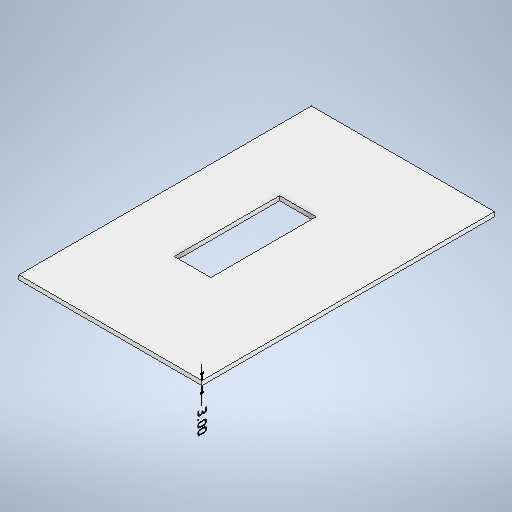
# Autodesk Inventor part: Q top 2
Saved by Autodesk Inventor 2025.3 (Build 293356000, 356)
## iProperties
Created: 2026-04-17
Part Number: Q top 2
Material: ABS Plastic
Document SubType Name: Modeling
Designer: logien
Density: 1.06 g/cm^3
Appearance: Smooth - White
Author: logien
Autodesk Inventor part; units mm, degrees
ref_plane "YZ Plane" through (0, 0, 0) normal (1, 0, 0) x (0, 1, 0)
ref_plane "XZ Plane" through (0, 0, 0) normal (0, 1, 0) x (-1, 0, 0)
ref_plane "XY Plane" through (0, 0, 0) normal (0, 0, 1) x (1, 0, 0)
sketch "Sketch1" plane through (0, 0, 0) normal (0, 1, 0) x (-1, 0, 0)
  line L0 (0, 0) -> (125.16, 0)
  line L1 (125.16, 0) -> (125.16, -200)
  line L2 (125.16, -200) -> (0, -200)
  line L3 (0, -200) -> (0, 0)
  dimension "d0" = 200
  dimension "d1" = 125.16
  constraints: 8 end point, 2 parallel, 1 horizontal, 1 perpendicular
  measures "d0" distance of L2.end L0.start
  measures "d1" distance of L0.start L0.end
extrude "Extrusion1" add sketch "Sketch1" along normal blind 3
sketch "Sketch2" plane through (0, 3, 0) normal (0, 1, 0) x (1, 0, 0)
  line L0 (-82.935, 64) -> (-57.935, 64)
  line L1 (-57.935, 64) -> (-57.935, 136)
  line L2 (-57.935, 136) -> (-82.935, 136)
  line L3 (-82.935, 136) -> (-82.935, 64)
  line L4 (-125.16, 200) -> (-125.16, 0) projected
  line L5 (0, 200) -> (-125.16, 200) projected
  point P0 (0, 0)
  dimension "d4" = 72
  dimension "d5" = 25
  dimension "d6" = 42.225
  dimension "d7" = 64
  constraints: 8 end point, 2 parallel, 1 horizontal, 1 perpendicular
  measures "d4" distance of L2.end L0.start
  measures "d5" distance of L0.start L0.end
  measures "d6" distance between parallel lines of L4 L3
  measures "d7" distance between parallel lines of L5 L2
extrude "Extrusion2" cut sketch "Sketch2" against normal blind 3
body "Solid1"
